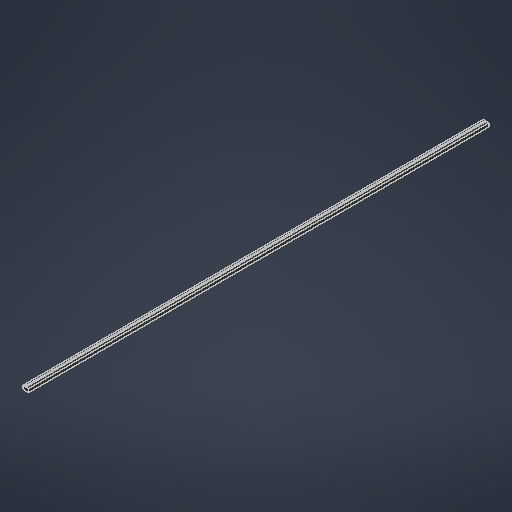
# Autodesk Inventor part: SP40-04A JUNTA INT CRISTAL ZOCALO 602 mm
Saved by Autodesk Inventor 2025 (Build 290162000, 162)
## iProperties
Created: 2026-01-20
Part Number: SP40-04A JUNTA INT CRISTAL ZOCALO 602 mm
Material: Caucho
Document SubType Name: Modeling
Designer: ROLANDO
Density: 0.93 g/cm^3
Appearance: Caucho - Negro
Author: ROLANDO
Autodesk Inventor part; units mm, degrees
ref_plane "YZ Plane" through (0, 0, 0) normal (1, 0, 0) x (0, 1, 0)
ref_plane "XZ Plane" through (0, 0, 0) normal (0, 1, 0) x (-1, 0, 0)
ref_plane "XY Plane" through (0, 0, 0) normal (0, 0, 1) x (1, 0, 0)
sketch "Boceto1" plane through (0, 0, 0) normal (0, 0, 1) x (1, 0, 0)
  line L0 (2.2697, 4.9951) -> (-0.1303, 4.9951)
  line L1 (-0.1303, 4.9951) -> (-0.1303, 0.1843)
  line L2 (2.2697, 4.9951) -> (2.2697, 3.7451)
  line L3 (2.2697, 3.7451) -> (2.9755, 3.7451)
  line L4 (2.9755, 3.7451) -> (3.6697, 4.7551)
  line L5 (-0.1303, 0.1843) -> (7.1697, 0.1843)
  line L6 (7.1697, 4.7551) -> (7.1697, 0.1843)
  line L7 (7.1697, 4.7551) -> (3.6697, 4.7551)
  dimension "d93" = 4.8108
  dimension "d94" = 0.24
  dimension "d95" = 2.4
  dimension "d96" = 0.7058
  dimension "d97" = 1.25
  dimension "d98" = 1.01
  dimension "d99" = 124.5
  dimension "d100" = 7.3
  constraints: 16 end point, 1 horizontal, 1 vertical
  measures "d93" distance of L0.end L1.end
  measures "d94" distance between parallel lines of L7 L0
  measures "d95" distance of L0.start L0.end
  measures "d96" distance of L2.end L4.start
  measures "d97" distance of L0.start L2.end
  measures "d98" vertical distance of L4.start L4.end
  measures "d99" angle of L3 L4
  measures "d100" distance between parallel lines of L6 L1
extrude "Extrusión1" add sketch "Boceto1" against normal blind 602
